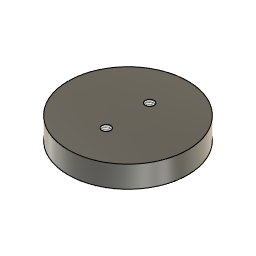
roud v1 (Autodesk Fusion 360 design; units mm, degrees)
Autodesk Fusion 360 part; units mm, degrees
sketch "草图1" plane through (0, 0, 0) normal (0, 0, 1) x (1, 0, 0)
  circle A0 centre (0, 0) radius 11
  dimension "d1" = 22
  constraint coincident A0.centre origin
  measures "d1" diameter of A0
extrude "拉伸1" add sketch "草图1" along normal blind 4
hole "孔1" at (0, 0, 4) direction (0, 0, -1) diameter 1.623 depth 10 tip angle 180
thread "螺纹1" "ISO Metric profile 2.0 M2x0.4 6H" thread offset 0 thread depth 10
move_face "MoveFace1" to x (1, 0, 0) y (0, 1, 0) z (0, 0, 1) at (0, -4, 0) 1 faces at (0.0808, -0.8075, 2.6667)
hole "孔2" at (0, 0, 4) direction (0, 0, -1) diameter 1.623 depth 10 tip angle 180
thread "螺纹2" "ISO Metric profile 2.0 M2x0.4 6H" thread offset 0 thread depth 10
move_face "MoveFace2" to x (1, 0, 0) y (0, 1, 0) z (0, 0, 1) at (0, 4, 0) 1 faces at (0.0808, -0.8075, 2.6667)
